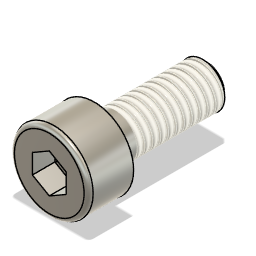
EchoWeather_Main (Autodesk Fusion 360 archive; units mm, degrees)
design "Broached Hexagon Socket Head Cap Screw ASME B18.3.1M - M4x0.7 x 10 Steel Grade 2 Plain"
description: Broached Hexagon Socket Head Cap Screw ASME B18.3.1M - M4x0.7 x 10
part number: BSHCS ASME B18.3.1M - M4x0.7 x 10 Steel Grade 2 Plain
Autodesk Fusion 360 part; units mm, degrees
sketch "Sketch1" plane through (0, 0, 0) normal (0, 1, 0) x (1, 0, 0)
  line L0 (-2, 0) -> (-2, 10)
  line L1 (-2, 10) -> (0, 10)
  line L2 (0, 10) -> (0, -4)
  line L3 (-2, 0) -> (-3.5, 0)
  line L4 (-3.5, 0) -> (-3.5, -4)
  line L5 (-3.5, -4) -> (0, -4)
  dimension "d9" = 4
  dimension "d66" = 7
  dimension "d101" = 10
  dimension "d102" = 4
  constraint perpendicular L0 L1
  constraint collinear origin L1.end L2.end
  constraint perpendicular L0 L3
  constraint coincident origin L3
  constraint vertical L0
  constraint vertical L2
  constraint parallel L2 L4
  constraint coincident L2 L5.end
  constraint perpendicular L2 L5
  measures "d101" distance of origin L1
  measures "d102" distance of L3.end L5
revolve "Revolve1" add sketch "Sketch1" angle 360 about axis through (0, 0, -10) along (0, 0, 1)
ref_plane "WorkPlane1" through (0, 0, 4) normal (0, 0, 1) x (1, 0, 0)
sketch "Sketch6" plane through (0, 0, 4) normal (0, 0, 1) x (1, 0, 0)
  line L0 (-1.5, 0) -> (1.5, 0) construction
  line L1 (0, 0) -> (-1.5, 0.866)
  line L2 (-1.5, -0.866) -> (-1.5, 0.866)
  line L3 (-1.5, -0.866) -> (0, 0)
  dimension "d100" = 150
  dimension "d103" = 3
  constraint horizontal L0
  constraint midpoint L1.start L0
  constraint coincident L1.start L3.end
  constraint perpendicular L0 L2
  constraint midpoint L0.start L2
  constraint coincident L1.end L2.end
  measures "d100" angle of L0 L1
  measures "d103" distance of L0.end L2
extrude "Extrude1" cut sketch "Sketch6" against normal blind 2
pattern_circular "C-Pattern1" count 6 over 360 about axis through (0, 0, 1.75) along (0, 0, 1) of "Extrude1"
extrude "Extrude2" cut 1 faces at (0, -0.5774, 2) along direction (0, 0, -1) blind 2 draft -85
thread "Thread3" "ANSI Metric M Profile 4.0 M4x0.7 M4x0.7 4g6g" major diameter 3.908 minor diameter 3.128 pitch 0.7 angle 60 resizes the face on face at (-1.9901, 0.1991, -3.3333) from (0, 0, -1.8294) to (0, 0, -10)
fillet "Fillet4" radius 0.4 1 edges at (-3.2631, 1.2657, 4)
sketch "Sketch7" plane through (0, 0, 0) normal (0, 1, 0) x (1, 0, 0)
  line L0 (-2.04, 10) -> (-2.04, 9.5706)
  line L1 (-2.04, 9.5706) -> (-1.5706, 10)
  line L2 (0, 10) -> (0, -4)
  line L3 (-2.04, 10) -> (0, 10)
  dimension "d104" = 1.5706
  dimension "d105" = 2.04
  dimension "d106" = 0.4294
  constraint coincident L2.start L3.end
  constraint perpendicular L2 L3
  constraint coincident L1.end L3
  constraint perpendicular L0 L3
  measures "d104" distance of L1.end L2
  measures "d105" distance of L0 L2.start
  measures "d106" distance of L0.end L3
revolve "Revolve3" cut sketch "Sketch7" angle 360 about axis through (0, 0, 1.75) along (0, 0, 1)
equation "d9 = adsk_nomdia"
equation "adsk_nomlen = 10.00 mm"
equation "adsk_headh = 4.00 mm"
equation "adsk_headdia = 7.00 mm"
equation "adsk_nomdia = 4.00 mm"
equation "adsk_philwidth = 3.00 mm"
equation "d31 = -adsk_phildepth"
equation "adsk_phildepth = 2.00 mm"
equation "d66 = adsk_headdia"
equation "d71 = adsk_headh"
equation "d76 = -adsk_phildepth"
equation "adsk_thrlen = 8.170585 mm"
equation "d86 = adsk_nomdia * 0.1"
equation "adsk_startlen = 0.429415 mm"
equation "adsk_endpointdia = 3.14117 mm"
equation "d101 = adsk_nomlen"
equation "d102 = adsk_headh"
equation "d103 = adsk_philwidth"
equation "d104 = adsk_endpointdia / 2"
equation "d105 = adsk_nomdia * 0.51"
equation "d106 = adsk_startlen"
equation "d108 = min(adsk_thrlen; adsk_nomlen - 0.001 mm)"

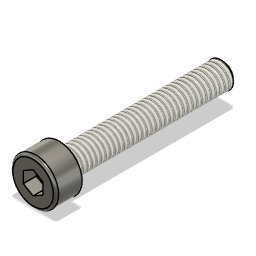
design "Broached Hexagon Socket Head Cap Screw ASME B18.3.1M - M4x0.7 x 25 Steel Grade 2 Plain"
description: Broached Hexagon Socket Head Cap Screw ASME B18.3.1M - M4x0.7 x 25
part number: BSHCS ASME B18.3.1M - M4x0.7 x 25 Steel Grade 2 Plain
Autodesk Fusion 360 part; units mm, degrees
sketch "Sketch1" plane through (0, 0, 0) normal (0, 1, 0) x (1, 0, 0)
  line L0 (-2, 0) -> (-2, 25)
  line L1 (-2, 25) -> (0, 25)
  line L2 (0, 25) -> (0, -4)
  line L3 (-2, 0) -> (-3.5, 0)
  line L4 (-3.5, 0) -> (-3.5, -4)
  line L5 (-3.5, -4) -> (0, -4)
  dimension "d9" = 4
  dimension "d66" = 7
  dimension "d101" = 25
  dimension "d102" = 4
  constraint perpendicular L0 L1
  constraint collinear origin L1.end L2.end
  constraint perpendicular L0 L3
  constraint coincident origin L3
  constraint vertical L0
  constraint vertical L2
  constraint parallel L2 L4
  constraint coincident L2 L5.end
  constraint perpendicular L2 L5
  measures "d101" distance of origin L1
  measures "d102" distance of L3.end L5
revolve "Revolve1" add sketch "Sketch1" angle 360 about axis through (0, 0, -25) along (0, 0, 1)
ref_plane "WorkPlane1" through (0, 0, 4) normal (0, 0, 1) x (1, 0, 0)
sketch "Sketch6" plane through (0, 0, 4) normal (0, 0, 1) x (1, 0, 0)
  line L0 (-1.5, 0) -> (1.5, 0) construction
  line L1 (0, 0) -> (-1.5, 0.866)
  line L2 (-1.5, -0.866) -> (-1.5, 0.866)
  line L3 (-1.5, -0.866) -> (0, 0)
  dimension "d100" = 150
  dimension "d103" = 3
  constraint horizontal L0
  constraint midpoint L1.start L0
  constraint coincident L1.start L3.end
  constraint perpendicular L0 L2
  constraint midpoint L0.start L2
  constraint coincident L1.end L2.end
  measures "d100" angle of L0 L1
  measures "d103" distance of L0.end L2
extrude "Extrude1" cut sketch "Sketch6" against normal blind 2
pattern_circular "C-Pattern1" count 6 over 360 about axis through (0, 0, 1.75) along (0, 0, 1) of "Extrude1"
extrude "Extrude2" cut 1 faces at (0, -0.5774, 2) along direction (0, 0, -1) blind 2 draft -85
thread "Thread3" "ANSI Metric M Profile 4.0 M4x0.7 M4x0.7 4g6g" major diameter 3.908 minor diameter 3.128 pitch 0.7 angle 60 resizes the face on face at (-1.9975, 0.0997, -8.3333) from (0, 0, -1.2588) to (0, 0, -25)
fillet "Fillet4" radius 0.4 1 edges at (-3.2631, 1.2657, 4)
sketch "Sketch7" plane through (0, 0, 0) normal (0, 1, 0) x (1, 0, 0)
  line L0 (-2.04, 25) -> (-2.04, 24.5706)
  line L1 (-2.04, 24.5706) -> (-1.5706, 25)
  line L2 (0, 25) -> (0, -4)
  line L3 (-2.04, 25) -> (0, 25)
  dimension "d104" = 1.5706
  dimension "d105" = 2.04
  dimension "d106" = 0.4294
  constraint coincident L2.start L3.end
  constraint perpendicular L2 L3
  constraint coincident L1.end L3
  constraint perpendicular L0 L3
  measures "d104" distance of L1.end L2
  measures "d105" distance of L0 L2.start
  measures "d106" distance of L0.end L3
revolve "Revolve3" cut sketch "Sketch7" angle 360 about axis through (0, 0, 1.75) along (0, 0, 1)
equation "d9 = adsk_nomdia"
equation "adsk_nomlen = 25.00 mm"
equation "adsk_headh = 4.00 mm"
equation "adsk_headdia = 7.00 mm"
equation "adsk_nomdia = 4.00 mm"
equation "adsk_philwidth = 3.00 mm"
equation "d31 = -adsk_phildepth"
equation "adsk_phildepth = 2.00 mm"
equation "d66 = adsk_headdia"
equation "d71 = adsk_headh"
equation "d76 = -adsk_phildepth"
equation "adsk_thrlen = 23.74117 mm"
equation "d86 = adsk_nomdia * 0.1"
equation "adsk_startlen = 0.429415 mm"
equation "adsk_endpointdia = 3.14117 mm"
equation "d101 = adsk_nomlen"
equation "d102 = adsk_headh"
equation "d103 = adsk_philwidth"
equation "d104 = adsk_endpointdia / 2"
equation "d105 = adsk_nomdia * 0.51"
equation "d106 = adsk_startlen"
equation "d108 = min(adsk_thrlen; adsk_nomlen - 0.001 mm)"
